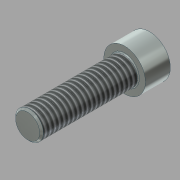
# Autodesk Inventor part: Hex Socket Screw
Saved by Autodesk Inventor 2011 SP2 (Build 150309200, 309)
## iProperties
Created: 2014-12-18
Part Number: Hex Socket Screw
Document SubType Name: Modeling
Designer: Greg Pavlik
Density: 1 g/cm^3
Author: Greg Pavlik
Autodesk Inventor part; units mm, degrees
ref_plane "YZ Plane" through (0, 0, 0) normal (1, 0, 0) x (0, 1, 0)
ref_plane "XZ Plane" through (0, 0, 0) normal (0, 1, 0) x (-1, 0, 0)
ref_plane "XY Plane" through (0, 0, 0) normal (0, 0, 1) x (1, 0, 0)
sketch "Sketch1" plane through (0, 0, 0) normal (0, 0, 1) x (1, 0, 0)
  line L0 (0, 0) -> (0, 10.8481)
  line L1 (0, 10.8481) -> (1.5, 11.25)
  line L2 (1.5, 11.25) -> (1.5, 13.5)
  line L3 (1.5, 13.5) -> (1.7304, 13.5)
  line L4 (2.25, 13.2) -> (2.25, 10.5)
  line L5 (2.25, 10.5) -> (1.5, 10.5)
  line L6 (1.5, 10.5) -> (1.5, 0)
  line L7 (1.5, 0) -> (0, 0)
  line L8 (1.7304, 13.5) -> (2.25, 13.2)
  dimension "Diameter" = 3
  dimension "d1" = 4.5
  dimension "d2" = 3
  dimension "Length" = 10.5
  dimension "d5" = 3
  dimension "d6" = 2.25
  dimension "d7" = 0.3
  dimension "d8" = 30
  dimension "d9" = 15
  constraints: 18 end point, 5 parallel, 1 perpendicular, 1 vertical
  measures "Diameter" diameter of L6 L0
  measures "d1" diameter of L4 L0
  measures "d2" distance between parallel lines of L5 L3
  measures "Length" distance between parallel lines of L7 L5
  measures "d5" diameter of L2 L0
  measures "d6" distance from line of L1.end L3
  measures "d7" distance from line of L4.start L3
  measures "d8" angle of L3 L8
  measures "d9" angle of L5 L1
revolve "Revolution1" add sketch "Sketch1" angle 360 about axis through (0, 0, 0) along (0, 1, 0)
sketch "Sketch2" plane through (0, 13.5, 0) normal (0, 1, 0) x (1, 0, 0)
  circle A0 centre (0, 0) radius 1.5 projected
  line L0 (0, -1.299) -> (-1.125, -0.6495)
  line L1 (-1.125, -0.6495) -> (-1.125, 0.6495)
  line L2 (-1.125, 0.6495) -> (0, 1.299)
  line L3 (0, 1.299) -> (1.125, 0.6495)
  line L4 (1.125, 0.6495) -> (1.125, -0.6495)
  line L5 (1.125, -0.6495) -> (0, -1.299)
  dimension "d14" = 2.25
  constraints: 12 end point, 1 coincident, 1 vertical, 13 other
  measures "d14" distance between parallel lines of L1 L4
extrude "Extrusion1" add sketch "Sketch2" against normal up to next
thread "Thread2" size "M3x0.5" class "6g" standard "ANSI Metric M Profile" full length
chamfer "Chamfer2" distance 0.2 angle 45 1 edges at (-1.5, 0, 0)
fillet "Fillet1" radius 0.1 1 edges at (-1.5, 10.5, 0)
equation "\"d1\" = 1.5 * Diameter"
equation "\"d2\" = Diameter"
equation "\"d5\" = Diameter"
equation "\"d6\" = 0.75 * Diameter"
equation "\"d7\" = 0.1 * Diameter"
equation "\"d14\" = 0.75 * Diameter"
body "Solid1"
